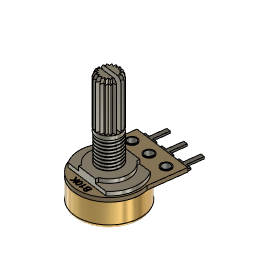
PotentiometerB10K (Autodesk Fusion 360 design; units mm, degrees)
Autodesk Fusion 360 part; units mm, degrees
sketch "Shaft" plane through (0, 0, 0) normal (0, 0, 1) x (1, 0, 0)
  circle A0 centre (0, 0) radius 2.25 construction
  circle A1 centre (0, 0) radius 3
  line L0 (0, 0) -> (0, 3) construction
  line L1 (0, 0) -> (0, 0.0849) construction
  line L2 (0, 0) -> (-0.3907, 2.2158) construction
  line L3 (0, 0) -> (0.3907, 2.2158) construction
  line L4 (-0.3907, 2.2158) -> (0, 3)
  line L5 (0.3907, 2.2158) -> (0, 3)
  line L6 (-0.3907, 2.2158) -> (-1.0261, 2.8191)
  line L7 (-1.125, 1.9486) -> (-1.0261, 2.8191)
  line L8 (-1.125, 1.9486) -> (-1.9284, 2.2981)
  line L9 (-1.7236, 1.4463) -> (-1.9284, 2.2981)
  line L10 (-1.7236, 1.4463) -> (-2.5981, 1.5)
  line L11 (-2.1143, 0.7695) -> (-2.5981, 1.5)
  line L12 (-2.1143, 0.7695) -> (-2.9544, 0.5209)
  line L13 (-2.25, 0) -> (-2.9544, 0.5209)
  line L14 (-2.25, 0) -> (-2.9544, -0.5209)
  line L15 (-2.1143, -0.7695) -> (-2.9544, -0.5209)
  line L16 (-2.1143, -0.7695) -> (-2.5981, -1.5)
  line L17 (-1.7236, -1.4463) -> (-2.5981, -1.5)
  line L18 (-1.7236, -1.4463) -> (-1.9284, -2.2981)
  line L19 (-1.125, -1.9486) -> (-1.9284, -2.2981)
  line L20 (-1.125, -1.9486) -> (-1.0261, -2.8191)
  line L21 (-0.3907, -2.2158) -> (-1.0261, -2.8191)
  line L22 (-0.3907, -2.2158) -> (0, -3)
  line L23 (0.3907, -2.2158) -> (0, -3)
  line L24 (0.3907, -2.2158) -> (1.0261, -2.8191)
  line L25 (1.125, -1.9486) -> (1.0261, -2.8191)
  line L26 (1.125, -1.9486) -> (1.9284, -2.2981)
  line L27 (1.7236, -1.4463) -> (1.9284, -2.2981)
  line L28 (1.7236, -1.4463) -> (2.5981, -1.5)
  line L29 (2.1143, -0.7695) -> (2.5981, -1.5)
  line L30 (2.1143, -0.7695) -> (2.9544, -0.5209)
  line L31 (2.25, 0) -> (2.9544, -0.5209)
  line L32 (2.25, 0) -> (2.9544, 0.5209)
  line L33 (2.1143, 0.7695) -> (2.9544, 0.5209)
  line L34 (2.1143, 0.7695) -> (2.5981, 1.5)
  line L35 (1.7236, 1.4463) -> (2.5981, 1.5)
  line L36 (2.958, 0.5) -> (-2.958, 0.5)
  line L37 (-2.958, -0.5) -> (2.958, -0.5)
  line L38 (1.7236, 1.4463) -> (1.9284, 2.2981)
  line L39 (1.125, 1.9486) -> (1.9284, 2.2981)
  line L40 (1.125, 1.9486) -> (1.0261, 2.8191)
  line L41 (0.3907, 2.2158) -> (1.0261, 2.8191)
  line L42 (0, 0) -> (3, 0) construction
  dimension "d109" = 4.5
  dimension "d110" = 6
  dimension "d111" = 20
  dimension "d113" = 360
  dimension "d114" = 1
  constraint coincident A0.centre A1.centre
  constraint concentric A0 A1
  constraint coincident A1 L0.end
  constraint vertical L0
  constraint coincident L0 L1.end
  constraint coincident A0 L2.end
  constraint coincident A0 L3.end
  constraint symmetric L0 L2 L3
  constraint coincident A1 L36.start
  constraint coincident A1 L36.end
  constraint coincident A1 L37.end
  constraint parallel L36 L37
  constraint coincident A1 L37.start
  constraint coincident A1 L42.end
  constraint horizontal L42
  constraint symmetric L36 L37 L42
  measures "d109" diameter of A0
  measures "d110" diameter of A1
  measures "d111" angle of L2 L3
  measures "d114" distance of L36 L37
extrude "Extrude1" add sketch "Shaft" along normal blind 1 makes body 1
extrude "Extrude2" add sketch "Shaft" along normal blind 12 from surface at 1 contours L4 L5 L6 L7 L8 L9 L10 L11 L12 L13 L32 L33 L34 L35 L36 L38 L39 L40 L41 | L14 L15 L16 L17 L18 L19 L20 L21 L22 L23 L24 L25 L26 L27 L28 L29 L30 L31 L37 bodies 1
chamfer "Chamfer1" distance 0.2 distance2 1 32 edges at (-2.5344, 0.6452, 13) (-2.3562, 1.1348, 13) (-2.1608, 1.4731, 13) (-1.826, 1.8722, 13) (-1.5267, 2.1233, 13) (-1.0755, 2.3838, 13) (-0.7084, 2.5174, 13) (-0.1954, 2.6079, 13) (0.1954, 2.6079, 13) (0.7084, 2.5174, 13) (1.0755, 2.3838, 13) (1.5267, 2.1233, 13) (1.826, 1.8722, 13) (2.1608, 1.4731, 13) (2.3562, 1.1348, 13) (2.5344, 0.6452, 13) (2.5344, -0.6452, 13) (2.3562, -1.1348, 13) (2.1608, -1.4731, 13) (1.826, -1.8722, 13) (1.5267, -2.1233, 13) (0.7084, -2.5174, 13) (1.0755, -2.3838, 13) (0.1954, -2.6079, 13) (-0.1954, -2.6079, 13) (-0.7084, -2.5174, 13) (-1.0755, -2.3838, 13) (-1.5267, -2.1233, 13) (-1.826, -1.8722, 13) (-2.1608, -1.4731, 13) (-2.3562, -1.1348, 13) (-2.5344, -0.6452, 13) measured on face at (0.1302, 1.7028, 13) measured on face at (0.1302, 1.7028, 13) measured on face at (0.1302, 1.7028, 13) measured on face at (0.1302, 1.7028, 13) measured on face at (0.1302, 1.7028, 13) measured on face at (0.1302, 1.7028, 13) measured on face at (0.1302, 1.7028, 13) measured on face at (0.1302, 1.7028, 13) measured on face at (0.1302, 1.7028, 13) measured on face at (0.1302, 1.7028, 13) measured on face at (0.1302, 1.7028, 13) measured on face at (0.1302, 1.7028, 13) measured on face at (0.1302, 1.7028, 13) measured on face at (0.1302, 1.7028, 13) measured on face at (0.1302, 1.7028, 13) measured on face at (0.1302, 1.7028, 13) measured on face at (-0.375, -1.1625, 13) measured on face at (-0.375, -1.1625, 13) measured on face at (-0.375, -1.1625, 13) measured on face at (-0.375, -1.1625, 13) measured on face at (-0.375, -1.1625, 13) measured on face at (-0.375, -1.1625, 13) measured on face at (-0.375, -1.1625, 13) measured on face at (-0.375, -1.1625, 13) measured on face at (-0.375, -1.1625, 13) measured on face at (-0.375, -1.1625, 13) measured on face at (-0.375, -1.1625, 13) measured on face at (-0.375, -1.1625, 13) measured on face at (-0.375, -1.1625, 13) measured on face at (-0.375, -1.1625, 13) measured on face at (-0.375, -1.1625, 13) measured on face at (-0.375, -1.1625, 13) on bodies 1
sketch "ScrewBase" plane through (0, 0, 0) normal (0, 0, 1) x (1, 0, 0)
  circle A0 centre (0, 0) radius 3
  circle A1 centre (0, 0) radius 5
  line L0 (-2.5, 4.3301) -> (-2.5, 5)
  line L1 (-2.5, 5) -> (2.5, 5)
  line L2 (2.5, 5) -> (2.5, 4.3301)
  line L3 (0, 0) -> (0, 5) construction
  line L4 (-2.5, -4.3301) -> (-2.5, -4.6099)
  line L5 (-2.5, -4.6099) -> (-2.5, -5)
  line L6 (-2.5, -5) -> (2.5, -5)
  line L7 (2.5, -5) -> (2.5, -4.3301)
  arc A2 (5.5902, -5) -> (5.5902, 5) centre (0, 0) ccw
  line L8 (2.5, 5) -> (5.5902, 5)
  line L9 (2.5, -5) -> (5.5902, -5)
  arc A3 (-5.5902, 5) -> (-5.5902, -5) centre (0, 0) ccw
  line L10 (-2.5, 5) -> (-5.5902, 5)
  line L11 (-2.5, -5) -> (-5.5902, -5)
  dimension "d120" = 6
  dimension "d123" = 10
  dimension "d124" = 5
  dimension "d125" = 7.5
  constraint coincident A0.centre A1.centre
  constraint coincident A1 L0.start
  constraint vertical L0
  constraint perpendicular L0 L1
  constraint coincident A1 L2.end
  constraint perpendicular L1 L2
  constraint midpoint L1 L3.end
  constraint vertical L3
  constraint tangent A1 L1
  constraint coincident A1 L4.start
  constraint vertical L4
  constraint parallel L4 L5
  constraint perpendicular L5 L6
  constraint coincident A1 L7.end
  constraint perpendicular L6 L7
  constraint collinear L2 L7
  constraint collinear L0 L5
  constraint tangent A1 L6
  constraint horizontal L8
  constraint horizontal L9
  constraint symmetric L1.end L3 L0.end
  constraint symmetric L3 L6.end L5.end
  constraint symmetric L3 A2.start A3.end
  constraint symmetric L3 A2.end A3.start
  constraint symmetric L3 A2 A3
  measures "d120" diameter of A0
  measures "d123" diameter of A1
  measures "d124" distance of L0.end L1.end
  measures "d125" radius of A2
extrude "Extrude3" add sketch "ScrewBase" against normal blind 7 separate body contours A0 makes body 2
thread "Thread1" "ISO Metric profile 6.0 M6x0.75 6g" major diameter 5.908 minor diameter 5.0475 pitch 0.75 angle 60 modelled right hand crest width 0.1053 on face at (2.9851, -0.2987, -4.6667) crest through (2.954, 0, 0.1875) on bodies 2
extrude "Extrude4" add sketch "ScrewBase" against normal blind 1 from surface at -7 contours A0 | A1 | A1 L1 L2 | A1 L6 L7 | A1 L0 L1 | A1 L4 L5 L6 bodies 2
extrude "Extrude5" add sketch "ScrewBase" against normal blind 1 from surface at -8 contours A0 | A1 | A1 L2 L7 A2 L8 L9 | A1 L1 L2 | A1 L6 L7 | A1 L0 L1 | A1 L4 L5 L6 | A1 L0 L4 L5 A3 L10 L11 bodies 2
sketch "Board" plane through (0, 0, -9) normal (0, 0, -1) x (1, 0, 0)
  arc A0 (5.5902, -5) -> (5.5902, 5) centre (0, 0) ccw construction
  line L0 (5.5902, 5) -> (-5.5902, 5) construction
  arc A1 (-5.5902, 5) -> (-5.5902, -5) centre (0, 0) ccw construction
  line L1 (-5.5902, -5) -> (5.5902, -5) construction
  circle A2 centre (0, 0) radius 8 construction
  line L2 (0, 0) -> (0, 8) construction
  line L3 (-7.5, -2.7839) -> (-7.5, -12)
  line L4 (-7.5, -12) -> (7.5, -12)
  line L5 (7.5, -12) -> (7.5, -2.7839)
  circle A3 centre (-5, -9) radius 1.25
  circle A4 centre (0, -9) radius 1.25
  circle A5 centre (5, -9) radius 1.25
  line L6 (-5, -9) -> (0, -9) construction
  line L7 (0, -9) -> (5, -9) construction
  arc A6 (7.5, -2.7839) -> (-7.5, -2.7839) centre (0, 0) ccw
  dimension "d132" = 16
  dimension "d133" = 15
  dimension "d134" = 20
  dimension "d135" = 2.5
  dimension "d136" = 2.5
  dimension "d137" = 3
  constraint coincident A0.centre A1.centre
  constraint coincident A2 L2.end
  constraint perpendicular L0 L2
  constraint coincident A2 L3.start
  constraint vertical L3
  constraint perpendicular L3 L4
  constraint coincident A2 L5.end
  constraint perpendicular L4 L5
  constraint equal A4 A5
  constraint equal A3 A4
  constraint coincident A3.centre L6.start
  constraint coincident A4.centre L6.end
  constraint coincident A5.centre L7.end
  constraint horizontal L7
  constraint equal L6 L7
  constraint horizontal L6
  constraint coincident L2 A4.centre
  measures "d132" diameter of A2
  measures "d133" distance of L3.end L4.end
  measures "d134" distance of L2.end L4
  measures "d135" diameter of A3
  measures "d136" distance of L3 A3.centre
  measures "d137" distance of L4 A3.centre
extrude "Extrude6" add sketch "Board" along normal blind 1 separate body makes body 3
sketch "B10K" plane through (0, 0, -9) normal (0, 0, 1) x (-1, 0, 0)
  circle A0 centre (-5, -9) radius 1.25
  circle A1 centre (0, -9) radius 1.25
  circle A2 centre (5, -9) radius 1.25
  arc A3 (7.5, -2.7839) -> (-7.5, -2.7839) centre (0, 0) ccw
  line L0 (-7.5, -2.7839) -> (-7.5, -12)
  line L1 (-7.5, -12) -> (7.5, -12)
  line L2 (7.5, -12) -> (7.5, -2.7839)
  line L3 (-2.3699, 5.6409) -> (2.3699, 5.6409) construction
  line L4 (2.3699, 5.6409) -> (2.3699, 7.6409) construction
  line L5 (2.3699, 7.6409) -> (-2.3699, 7.6409) construction
  line L6 (-2.3699, 7.6409) -> (-2.3699, 5.6409) construction
  line L7 (0, 0) -> (0, 0.5638) construction
  line L8 (0, 0.5638) -> (0, 7.6409) construction
  dimension "d141" = 2
  dimension "d142" = 4.7398
  text T0 "B10K" font "Arial" height 2 align ink ink in box 0 x 0 at (-2.3699, 5.6409) x (1, 0) y (0, 1) spacing 1 height is em
  constraint perpendicular L3 L4
  constraint parallel L3 L5
  constraint parallel L4 L6
  constraint coincident A3.centre L7.start
  constraint vertical L7
  constraint midpoint L5 L8.end
  constraint vertical L8
  constraint coincident A3 L4.end
  constraint coincident A3 L5.end
  measures "d141" distance of L3.end L4.end
  measures "d142" distance of L4.end L5.end
extrude "Extrude7" add sketch "B10K" along normal blind 0.01 text T0 bodies 3
sketch "Pin" plane through (0, 0, -10) normal (0, 0, -1) x (1, 0, 0)
  circle A0 centre (5, -9) radius 1.25 construction
  circle A1 centre (0, -9) radius 1.25 construction
  circle A2 centre (-5, -9) radius 1.25
  arc A3 (7.5, -2.7839) -> (-7.5, -2.7839) centre (0, 0) ccw construction
  line L0 (-7.5, -2.7839) -> (-7.5, -12) construction
  line L1 (-7.5, -12) -> (7.5, -12) construction
  line L2 (7.5, -12) -> (7.5, -2.7839) construction
  circle A4 centre (-5, -9) radius 1
  circle A5 centre (-5, -9) radius 1.75 construction
  line L3 (-5, -7.25) -> (-5, -13.25) construction
  line L4 (-6.75, -9) -> (-6.75, -13.25)
  line L5 (-3.25, -13.25) -> (-3.25, -9)
  line L6 (-4.5, -13.25) -> (-4.5, -17.25)
  line L7 (-4.5, -17.25) -> (-5.5, -17.25)
  line L8 (-5.5, -17.25) -> (-5.5, -13.25)
  arc A6 (-3.25, -9) -> (-6.75, -9) centre (-5, -9) ccw
  line L9 (-6.75, -13.25) -> (-5.5, -13.25)
  line L10 (-4.5, -13.25) -> (-3.25, -13.25)
  line L11 (-5, -13.25) -> (-5, -17.25) construction
  dimension "d145" = 2
  dimension "d146" = 3.5
  dimension "d147" = 6
  dimension "d148" = 4
  dimension "d149" = 1
  dimension "d178" = 0
  constraint concentric A2 A4
  constraint concentric A2 A5
  constraint coincident A5 L3.start
  constraint perpendicular L1 L3
  constraint coincident A2.centre L3
  constraint coincident A5 L4.start
  constraint perpendicular L1 L4
  constraint coincident A5 L5.end
  constraint tangent A5 L5
  constraint vertical L5
  constraint tangent A5 L4
  constraint vertical L6
  constraint horizontal L7
  constraint vertical L8
  constraint coincident A2.centre A4.centre
  constraint perpendicular L8 L9
  constraint perpendicular L5 L10
  constraint collinear L9 L10
  constraint coincident L3.end L9
  constraint midpoint L7 L11.end
  constraint perpendicular L7 L11
  measures "d145" diameter of A4
  measures "d146" diameter of A5
  measures "d147" distance of L3.start L3.end
  measures "d148" distance of L8.end L7.end
  measures "d149" distance of L6.end L7.end
extrude "Extrude8" add sketch "Pin" along normal blind 0.5 separate body contours A2 | L4 L5 L6 L7 L8 A6 L9 L10 makes body 4
extrude "Extrude9" add sketch "Pin" against normal blind 1.2 separate body contours A2 makes body 5
combine "Combine1" operation add target body 4 tool bodies 5
pattern_linear "R-Pattern1" count 3 spacing 5 along (1, 0, 0) of bodies 4 makes body 6 at (0.8718, 12.1436, -10.5) makes body 7 at (5.8718, 12.1436, -10.5)
sketch "Casing" plane through (0, 0, -10) normal (0, 0, -1) x (1, 0, 0)
  circle A0 centre (5, -9) radius 1.25
  circle A1 centre (0, -9) radius 1.25
  circle A2 centre (-5, -9) radius 1.25
  arc A3 (7.5, -2.7839) -> (-7.5, -2.7839) centre (0, 0) ccw
  line L0 (-7.5, -2.7839) -> (-7.5, -12)
  line L1 (-7.5, -12) -> (7.5, -12)
  line L2 (7.5, -12) -> (7.5, -2.7839)
  circle A4 centre (0, 0) radius 8
  dimension "d175" = 0
  dimension "d176" = 0
  dimension "d177" = 0
  constraint concentric A3 A4
extrude "Extrude10" add sketch "Casing" along normal blind 6 separate body contours A1 A4 | A1 A3 A4 picked at (-0.0278, -7.9153) makes body 8
fillet "Fillet1" radius 1 1 edges at (-7.4586, 2.8929, -16) on bodies 8
copy_body "Body->Comp1" bodies 1 removing the originals makes body 9 in component "Shaft"
copy_body "Body->Comp2" bodies 2 removing the originals makes body 10 in component "ScrewBase"
copy_body "Body->Comp3" bodies 3 removing the originals makes body 11 in component "Board"
copy_body "Body->Comp4" bodies 4 removing the originals makes body 12 in component "Pin1"
copy_body "Body->Comp5" bodies 6 removing the originals makes body 13 in component "Pin2"
copy_body "Body->Comp6" bodies 7 removing the originals makes body 14 in component "Pin3"
copy_body "Body->Comp7" bodies 8 removing the originals makes body 15 in component "Casing"
component "Shaft" placed x (0.991445, -0.130526, 0) y (0.130526, 0.991445, 0) z (0, 0, 1) at (34.5949, 33.1665, 10.6873)
component "ScrewBase" placed x (0.991445, -0.130526, 0) y (0.130526, 0.991445, 0) z (0, 0, 1) at (34.6057, 33.2494, 10.6873)
component "Board" placed x (0.991445, -0.130526, 0) y (0.130526, 0.991445, 0) z (0, 0, 1) at (34.6057, 33.2494, 10.6873)
component "Pin1" placed x (0.991445, -0.130526, 0) y (0.130526, 0.991445, 0) z (0, 0, 1) at (34.6057, 33.2494, 10.6873)
component "Pin2" placed x (0.991445, -0.130526, 0) y (0.130526, 0.991445, 0) z (0, 0, 1) at (34.6057, 33.2494, 10.6873)
component "Pin3" placed x (0.991445, -0.130526, 0) y (0.130526, 0.991445, 0) z (0, 0, 1) at (34.6057, 33.2494, 10.6873)
component "Casing" placed x (0.991445, -0.130526, 0) y (0.130526, 0.991445, 0) z (0, 0, 1) at (34.6057, 33.2494, 10.6873)
equation "d111 = ( 360 / 18 ) * 1 deg"
named bodies: "Shaft", "ScrewBase", "Board", "Pin1", "Pin2", "Pin3", "Casing"
